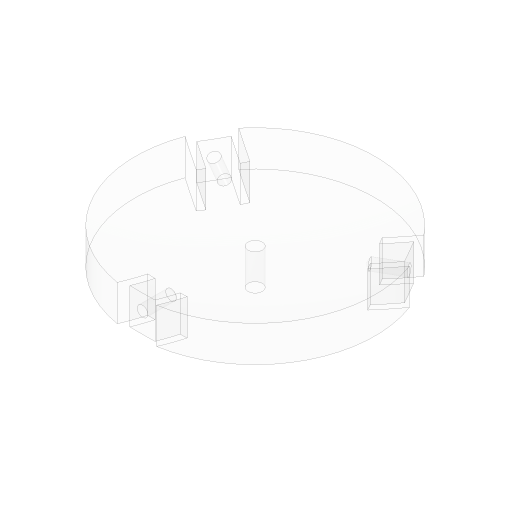
# Autodesk Inventor part: Parachute bulkhead
Saved by Autodesk Inventor 2024 (Build 280153000, 153)
## iProperties
Created: 2023-12-30
Part Number: Parachute bulkhead
Material: PET Plastic
Document SubType Name: Modeling
Designer: Jamie
Density: 1.541 g/cm^3
Appearance: Polycarbonate - Clear
Mass: 51.6308 g
Surface Area: 102.74 cm^2
Volume: 33.5047 cm^3
Author: Jamie
Autodesk Inventor part; units mm, degrees
ref_plane "YZ Plane" through (0, 0, 0) normal (1, 0, 0) x (0, 1, 0)
ref_plane "XY Plane" through (0, 0, 0) normal (0, 0, 1) x (1, 0, 0)
sketch "Sketch2" plane through (0, 0, 0) normal (1, 0, 0) x (0, 1, 0)
  arc A0 (15, 33.5) -> (10, 0) centre (124.725, 0) ccw construction
  arc A1 (5, 33.5) -> (0, 0) centre (114.725, 0) ccw construction
  line L0 (15, 33.5) -> (5, 33.5)
  line L1 (10, 0) -> (0, 0) construction
  line L2 (-26.4367, 0) -> (149.9186, 0) projected
  line L3 (10.0174, 2) -> (0.0174, 2)
  arc A2 (5, 33.5) -> (0.0174, 2) centre (114.725, 0) ccw
  arc A3 (15, 33.5) -> (10.0174, 2) centre (124.725, 0) ccw
  point P0 (0, 0)
  point P1 (15, 0)
  dimension "d6" = 5
  dimension "d8" = 10
  dimension "d10" = 10
  dimension "d12" = 2
  constraints: 11 point on circle, 6 end point, 4 centre point, 2 coincident, 2 horizontal
  measures "d6" horizontal distance of L1.end L0.end
  measures "d8" distance of L1.start point (0, 0)
  measures "d10" distance of L0.start L0.end
  measures "d12" distance between parallel lines of L1 L3
revolve "Revolution2" add sketch "Sketch2" angle 360 about axis through (0, -10, 0) along (0, 1, 0)
ref_plane "Work Plane2" through (0, 26.25, 0) normal (0, 1, 0) x (-1, 0, 0)
sketch "Sketch5" plane through (0, 26.25, 0) normal (0, 1, 0) x (-1, 0, 0)
  circle A0 centre (0, 0) radius 33.5 projected
  line L0 (-5.5, 33.0454) -> (5.5, 33.0454) construction
  line L1 (-5.5, 33.0454) -> (-5.5, 24.5)
  line L2 (-5.5, 24.5) -> (-3.5, 24.5)
  line L3 (-3.5, 24.5) -> (-3.5, 31.5)
  line L4 (-3.5, 31.5) -> (3.5, 31.5)
  line L5 (3.5, 31.5) -> (3.5, 24.5)
  line L6 (3.5, 24.5) -> (5.5, 24.5)
  line L7 (5.5, 24.5) -> (5.5, 33.0454)
  circle A1 centre (0, 0) radius 2 projected
  arc A2 (5.5, 33.0454) -> (-5.5, 33.0454) centre (0, 0) ccw
  line L8 (5.5, 33.0454) -> (0, 0) construction
  line L9 (0, 0) -> (0, 33.5) construction
  line L10 (5.5, 24.5) -> (0, 0) construction
  line L11 (6.965, 32.7679) -> (0, 0) construction
  line L12 (6.965, 32.7679) -> (6.5492, 30.8116) construction
  point P0 (0, 31.5)
  dimension "d37" = 11
  dimension "d40" = 2
  dimension "d41" = 2
  dimension "d56" = 9
  dimension "d57" = 2
  dimension "d58" = 33.0454
  dimension "d59" = 2
  dimension "d60" = 0
  dimension "d61" = 0
  dimension "d62" = 12
  constraints: 26 end point, 6 point on circle, 5 perpendicular, 3 point on line, 1 centre point, 1 coincident, 1 horizontal, 1 midpoint, 1 vertical
  measures "d37" distance of L0.start L0.end
  measures "d40" distance between parallel lines of L3 L1
  measures "d41" distance between parallel lines of L7 L5
  measures "d56" distance from line of L9.end L6
  measures "d57" distance of L9.end point (0, 31.5)
  measures "d58" distance from line of point (0, 0) L0
  measures "d59" distance of L11.start L12.end
  measures "d60" distance of point (0, 0) L11.end
  measures "d61" distance of A0.centre L11.end
  measures "d62" angle of L9 L11
extrude "Extrusion3" cut sketch "Sketch5" along normal through all both and the other way through all contours L7 L6 L5 L4 L3 L2 L1 A0 picked at (-4.8333, 29.6818)
sketch "Sketch6" plane through (0, 124.725, 31.5) normal (0, 0, 1) x (1, 0, 0)
  line L0 (33.5, -109.725) -> (-33.5, -109.725) projected
  point P0 (0, -124.725)
  point P1 (0, -114.725)
  point P2 (5.5, -109.725)
  point P3 (-5.5, -109.725)
  dimension "d45" = 5
  measures "d45" distance from line of point (0, -114.725) L0
hole "Hole2" at (0, 10, 31.5) direction (0, 0, -1) diameter 3 depth 8 tip angle 118
pattern_circular "Circular Pattern2" count 3 over 360 about axis through (0, 10, 0) along (0, 1, 0) of "Hole2", "Extrusion3"
body "Solid3"
